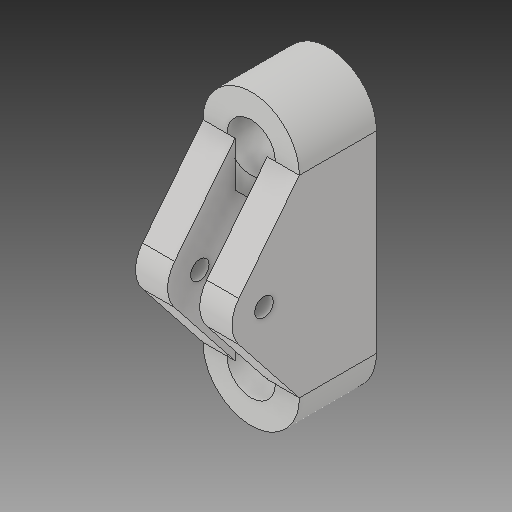
# Autodesk Inventor part: combo cross head
Saved by Autodesk Inventor 2017 SP1 (Build 210196100, 196)
## iProperties
Created: 2017-08-15
Part Number: combo cross head
Material: Generic
Document SubType Name: Modeling
Designer: zimirken
Density: 1 g/cm^3
Appearance: Default
Author: zimirken
Autodesk Inventor part; units mm, degrees
ref_plane "YZ Plane" through (0, 0, 0) normal (1, 0, 0) x (0, 1, 0)
ref_plane "XZ Plane" through (0, 0, 0) normal (0, 1, 0) x (-1, 0, 0)
ref_plane "XY Plane" through (0, 0, 0) normal (0, 0, 1) x (1, 0, 0)
sketch "Sketch1" plane through (0, 0, 0) normal (0, 0, 1) x (1, 0, 0)
  circle A0 centre (0, 0) radius 3.05
  line L0 (0, 30) -> (0, -30) construction
  circle A1 centre (0, 30) radius 7.5
  circle A2 centre (0, -30) radius 7.5
  line L1 (0, 30) -> (0, -30) construction
  line L2 (15, 30) -> (15, -30)
  line L3 (-15, -30) -> (-15, 30)
  arc A3 (15, 30) -> (-15, 30) centre (0, 30) ccw
  arc A4 (-15, -30) -> (15, -30) centre (0, -30) ccw
  point P0 (0, 0)
  dimension "d0" = 30
  dimension "d1" = 6.1
  dimension "d2" = 15
  dimension "d3" = 30
  constraints: 10 end point, 5 centre point, 4 coincident, 4 point on circle, 4 tangent, 2 equal length, 2 midpoint, 1 equal radius, 1 vertical
  measures "d0" distance of L0.start point (0, 0)
  measures "d1" diameter of A0
  measures "d2" diameter of A1
  measures "d3" distance between parallel lines of L2 L3
extrude "Extrusion1" add sketch "Sketch1" along normal blind 24
sketch "Sketch2" plane through (0, 0, 24) normal (0, 0, 1) x (1, 0, 0)
  circle A0 centre (0, -30) radius 7.5 construction
  circle A1 centre (0, 30) radius 7.5 construction
  circle A2 centre (0, 0) radius 3.05 construction
  line L0 (15, -30) -> (15, 30) construction
  arc A3 (15, 30) -> (-15, 30) centre (0, 30) ccw construction
  line L1 (-15, 30) -> (-15, -30) construction
  arc A4 (-15, -30) -> (15, -30) centre (0, -30) ccw construction
  line L2 (5, -16) -> (-5, -16)
  line L3 (-5, -16) -> (-5, 16)
  line L4 (-5, 16) -> (5, 16)
  line L5 (5, 16) -> (5, -16)
  line L6 (5, -16) -> (-5, 16) construction
  line L7 (-5, -16) -> (5, 16) construction
  dimension "d6" = 10
  dimension "d7" = 32
  constraints: 12 end point, 2 midpoint, 2 parallel, 1 horizontal, 1 perpendicular
  measures "d6" distance of L3.end L4.end
  measures "d7" distance of L2.end L3.end
extrude "Extrusion2" cut sketch "Sketch2" against normal blind 14
sketch "Sketch3" plane through (15, -30, 0) normal (1, 0, 0) x (0, 0, -1)
  line L0 (0, 60) -> (0, 0) construction
  line L1 (0, 60) -> (-24, 60) construction
  line L2 (-24, 0) -> (-24, 60) construction
  line L3 (0, 0) -> (-24, 0) construction
  line L4 (-24, 14) -> (-24, 46) construction
  line L5 (-24, 14) -> (-10, 14) construction
  line L6 (-10, 14) -> (-10, 46) construction
  line L7 (-24, 46) -> (-10, 46) construction
  line L8 (-24, 30) -> (-35, 30) construction
  circle A0 centre (-35, 30) radius 2.9
  arc A1 (-42.8398, 36.2079) -> (-42.8398, 23.7921) centre (-35, 30) ccw
  line L9 (-42.8398, 36.2079) -> (-24, 60)
  line L10 (-42.8398, 23.7921) -> (-24, 0)
  line L11 (-24, 60) -> (-24, 0)
  line L12 (-24, 52.5) -> (-24, 67.5) projected
  point P0 (0, 30)
  dimension "d10" = 25
  dimension "d11" = 5.8
  dimension "d12" = 10
  constraints: 8 end point, 2 centre point, 2 coincident, 2 point on circle, 2 tangent, 1 collinear, 1 horizontal, 1 midpoint
  measures "d10" distance from line of L8.end L6
  measures "d11" diameter of A0
  measures "d12" radius of A1
extrude "Extrusion3" add sketch "Sketch3" against normal up to surface (10 mm away)
mirror "Mirror1" about plane through (0, 0, 0) normal (1, 0, 0) of "Extrusion3"
body "Solid1"
